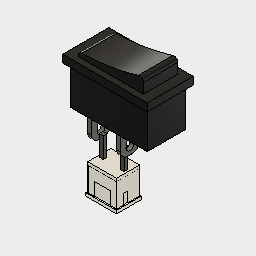
NewAssembly (Autodesk Fusion 360 archive; units mm, degrees)
design "Rocket Swith 15*10"
Autodesk Fusion 360 part; units mm, degrees
sketch "Sketch1" plane through (0, 0, 0) normal (0, 1, 0) x (1, 0, 0)
  line L0 (-10, 5) -> (10, 5)
  line L1 (10, 5) -> (10, -5)
  line L2 (10, -5) -> (-10, -5)
  line L3 (-10, -5) -> (-10, 5)
  dimension "d1" = 20
  dimension "d2" = 10
  dimension "d3" = 5
  dimension "d4" = 10
  measures "d1" distance of L0.start L0.end
  measures "d2" distance of L0.start L2.end
  measures "d3" distance of origin L0
  measures "d4" distance of origin L3
extrude "Extrude1" add sketch "Sketch1" along normal blind 10 makes body 1
sketch "Sketch2" plane through (0, 10, 0) normal (0, 1, 0) x (-1, 0, 0)
  line L0 (10, 5) -> (-10, 5)
  line L1 (-10, 5) -> (-10, -5)
  line L2 (-10, -5) -> (10, -5)
  line L3 (10, -5) -> (10, 5)
  line L4 (11, 6) -> (-11, 6)
  line L5 (-11, 6) -> (-11, -6)
  line L6 (-11, -6) -> (11, -6)
  line L7 (11, -6) -> (11, 6)
  dimension "d7" = 1
extrude "Extrude2" add sketch "Sketch2" along normal blind 2 contours L0 L1 L2 L3 | L4 L5 L6 L7 bodies 1
sketch "Sketch3" plane through (0, 12, 0) normal (0, 1, 0) x (-1, 0, 0)
  line L0 (11, -6) -> (11, 6)
  line L1 (11, 6) -> (-11, 6)
  line L2 (-11, 6) -> (-11, -6)
  line L3 (-11, -6) -> (11, -6)
  line L4 (-10, 5) -> (10, 5)
  line L5 (10, 5) -> (10, -5)
  line L6 (10, -5) -> (-10, -5)
  line L7 (-10, -5) -> (-10, 5)
  line L8 (-9.5, 4.5) -> (9.5, 4.5)
  line L9 (9.5, 4.5) -> (9.5, -4.5)
  line L10 (9.5, -4.5) -> (-9.5, -4.5)
  line L11 (-9.5, -4.5) -> (-9.5, 4.5)
  line L12 (9.5, -4.5) -> (8.5, -4.5)
  line L13 (8.5, -4.5) -> (8.5, 4.5)
  line L14 (8.5, 4.5) -> (9.5, 4.5)
  line L15 (9.5, 4.5) -> (9.5, -4.5)
  line L16 (-9.5, -4.5) -> (-8.5, -4.5)
  line L17 (-8.5, -4.5) -> (-8.5, 4.5)
  line L18 (-8.5, 4.5) -> (-9.5, 4.5)
  line L19 (-9.5, 4.5) -> (-9.5, -4.5)
  dimension "d14" = 0.5
  dimension "d15" = 1
  dimension "d16" = 1
  measures "d15" distance of L9.end L12.end
  measures "d16" distance of L10.end L16.end
extrude "Extrude3" add sketch "Sketch3" along normal blind 4 contours L8 L10 L13 L17 bodies 1
sketch "Sketch5" plane through (0, 0, 4.5) normal (0, 0, 1) x (1, 0, 0)
  line L0 (-8.5, 12) -> (8.5, 12)
  line L1 (8.5, 12) -> (8.5, 16)
  line L2 (8.5, 16) -> (-8.5, 16)
  line L3 (-8.5, 16) -> (-8.5, 12)
  spline S0 degree 5 poles (-8.5, 13.1583) (-8.1503, 13.1635) (-7.4519, 13.1784) (-6.4067, 13.2142) (-5.0183, 13.2895) (-3.2919, 13.4325) (-1.5755, 13.6289) (0.1301, 13.8829) (1.8245, 14.1971) (3.5081, 14.5689) (5.1818, 14.9942) (6.5133, 15.3737) (7.5081, 15.6789) (8.1697, 15.8915) (8.5, 16) knots 0 0 0 0 0 0 0.1 0.2 0.3 0.4 0.5 0.6 0.7 0.8 0.9 1 1 1 1 1 1
  line L4 (8.5, 12) -> (-8.5, 12)
  line L5 (-8.5, 12) -> (-8.5, 16)
  line L6 (-8.5, 16) -> (8.5, 16)
  line L7 (8.5, 16) -> (8.5, 12)
  point P0 (0.1376, 13.8996)
extrude "Extrude5" cut sketch "Sketch5" against normal blind 9 contours L2 L3 S0 L5 L6 bodies 1
fillet "Fillet1" radius 1 2 edges at (8.5, 16, 0) (-8.5, 13.1583, 0) on bodies 1
sketch "Sketch6" plane through (0, 0, 0) normal (0, -1, 0) x (1, 0, 0)
  line L0 (10, 5) -> (-10, 5)
  line L1 (-10, 5) -> (-10, -5)
  line L2 (-10, -5) -> (10, -5)
  line L3 (10, -5) -> (10, 5)
  line L4 (-8, 2.5) -> (-7, 2.5)
  line L5 (-7, 2.5) -> (-7, -2.5)
  line L6 (-7, -2.5) -> (-8, -2.5)
  line L7 (-8, -2.5) -> (-8, 2.5)
  line L8 (-0.5, 2.5) -> (0.5, 2.5)
  line L9 (0.5, 2.5) -> (0.5, -2.5)
  line L10 (0.5, -2.5) -> (-0.5, -2.5)
  line L11 (-0.5, -2.5) -> (-0.5, 2.5)
  dimension "d20" = 5
  dimension "d21" = 1
  dimension "d22" = 7
  dimension "d23" = 5
  dimension "d24" = 1
  dimension "d25" = 0.5
  dimension "d26" = 2.5
  measures "d20" distance of L4.start L6.end
  measures "d21" distance of L4.start L4.end
  measures "d22" distance of origin L5
  measures "d23" distance of L8.start L10.end
  measures "d24" distance of L8.start L8.end
  measures "d25" distance of origin L11
  measures "d26" distance of origin L8
extrude "Extrude6" add sketch "Sketch6" along normal blind 8 contours L4 L5 L6 L7 | L8 L9 L10 L11 bodies 1
sketch "Sketch7" plane through (0.5, 0, 0) normal (1, 0, 0) x (0, 0, -1)
  line L0 (2.5, 0) -> (-2.5, 0)
  line L1 (-2.5, 0) -> (-2.5, -8)
  line L2 (-2.5, -8) -> (2.5, -8)
  line L3 (2.5, -8) -> (2.5, 0)
  line L4 (1, -6) -> (1, -5)
  arc A0 (1, -5) -> (-1, -5) centre (0, -5) ccw
  line L5 (-1, -5) -> (-1, -6)
  arc A1 (-1, -6) -> (1, -6) centre (0, -6) ccw
  line L6 (0, -6) -> (0, -5) construction
  dimension "d29" = 1
  dimension "d30" = 1
  dimension "d31" = 5
  measures "d29" radius of A1
  measures "d30" distance of A1.centre A0.centre
  measures "d31" distance of origin A0.centre
extrude "Extrude7" cut sketch "Sketch7" against normal blind 8.5 contours L4 A0 L5 A1 bodies 1
fillet "Fillet2" radius 2 4 edges at (-7.5, -8, 2.5) (0, -8, 2.5) (0, -8, -2.5) (-7.5, -8, -2.5) on bodies 1
sketch "Sketch8" plane through (0, 0, -5) normal (0, 0, -1) x (-1, 0, 0)
  line L0 (-10, 0) -> (10, 0)
  line L1 (10, 0) -> (10, 10)
  line L2 (10, 10) -> (-10, 10)
  line L3 (-10, 10) -> (-10, 0)
  line L4 (7.5, -12) -> (0, -12)
  line L5 (0, -12) -> (0, -19)
  line L6 (0, -19) -> (7.5, -19)
  line L7 (7.5, -19) -> (7.5, -12)
  line L8 (6.5, -12) -> (7, -12)
  line L9 (7, -12) -> (7, -6)
  line L10 (7, -6) -> (6.5, -6)
  line L11 (6.5, -6) -> (6.5, -12)
  line L12 (0.5, -12) -> (1, -12)
  line L13 (1, -12) -> (1, -6)
  line L14 (1, -6) -> (0.5, -6)
  line L15 (0.5, -6) -> (0.5, -12)
  line L16 (0.5, 0) -> (0.5, -6)
  line L17 (7, 0) -> (7, -6)
  dimension "d35" = 7.5
  dimension "d36" = 7
  dimension "d37" = 12
  dimension "d38" = 0.5
  dimension "d39" = 0.5
  dimension "d40" = 6
  measures "d35" distance of L4.start L4.end
  measures "d36" distance of L4.start L6.end
  measures "d37" distance of origin L4
  measures "d38" distance of L13.end L14.end
  measures "d39" distance of L9.end L10.end
  measures "d40" distance of L8.end L9.end
extrude "Extrude8" add sketch "Sketch8" against normal blind 8 separate body contours L4 L5 L6 L7 L8 L12 makes body 2
extrude "Extrude9" cut 1 faces at (-2.8333, -16.6667, -5) along direction (0, 0, 1) blind 2 on bodies 2 bodies 2
sketch "Sketch9" plane through (0, -12, 0) normal (0, 1, 0) x (-1, 0, 0)
  line L0 (0, -3) -> (7.5, -3)
  line L1 (7.5, -3) -> (7.5, 3)
  line L2 (7.5, 3) -> (0, 3)
  line L3 (0, 3) -> (0, -3)
  line L4 (7, -0.5) -> (6, -0.5)
  line L5 (6, -0.5) -> (6, 0.5)
  line L6 (6, 0.5) -> (7, 0.5)
  line L7 (7, 0.5) -> (7, -0.5)
  line L8 (0.5, -0.5) -> (1.5, -0.5)
  line L9 (1.5, -0.5) -> (1.5, 0.5)
  line L10 (1.5, 0.5) -> (0.5, 0.5)
  line L11 (0.5, 0.5) -> (0.5, -0.5)
  line L12 (0.5, 1) -> (0.5, -1)
  line L13 (0.5, 1) -> (0.5, -1)
  line L14 (0.5, -0.5) -> (0.5, -2.5)
  line L15 (0.5, -0.5) -> (0.5, 0.5)
  line L16 (0.5, 2.5) -> (0.5, 0.5)
  line L17 (0.5, 2.5) -> (0.5, -2.5)
  line L18 (7, -2.5) -> (7, -0.5)
  line L19 (7, -2.5) -> (7, 2.5)
  line L20 (7, 0.5) -> (7, 2.5)
  line L21 (7, 0.5) -> (7, -0.5)
  line L22 (7, -1) -> (7, 1)
  line L23 (7, -1) -> (7, 1)
  point P0 (7, -2.5)
  dimension "d45" = 1
  dimension "d46" = 1
  dimension "d47" = 0.5
  dimension "d48" = 1
  measures "d45" distance of L8.start L8.end
  measures "d46" distance of L4.start L4.end
  measures "d47" distance of origin L8
  measures "d48" distance of L8.end L9.end
extrude "Extrude10" add sketch "Sketch9" along normal blind 5.326 contours L4 L5 L6 L7 L19 L21 L22 L23 | L8 L9 L10 L11 L12 L13 L15 L17 bodies 2
shell "Shell1" thickness 0.5 removed faces 1 at (-2.5, -19, -1) on bodies 2
sketch "Sketch10" plane through (0, 0, 0) normal (1, 0, 0) x (0, 0, -1)
  line L0 (3, -19) -> (3, -12)
  line L1 (3, -12) -> (-3, -12)
  line L2 (-3, -12) -> (-3, -19)
  line L3 (-3, -19) -> (3, -19)
  line L4 (-1.2673, -19) -> (0, -19)
  line L5 (0, -19) -> (0, -16.3604)
  line L6 (0, -16.3604) -> (-1.2673, -16.3604)
  line L7 (-1.2673, -16.3604) -> (-1.2673, -19)
extrude "Extrude11" cut sketch "Sketch10" against normal blind 7.5 contours L3 L4 L5 L6 L7 bodies 2
sketch "Sketch11" plane through (0, 0, 3) normal (0, 0, 1) x (1, 0, 0)
  line L0 (0, -19) -> (0, -12)
  line L1 (0, -12) -> (-7.5, -12)
  line L2 (-7.5, -12) -> (-7.5, -19)
  line L3 (-7.5, -19) -> (0, -19)
  line L4 (-5.8268, -19) -> (-1.5543, -19)
  line L5 (-1.5543, -19) -> (-1.5543, -15.6198)
  line L6 (-1.5543, -15.6198) -> (-5.8268, -15.6198)
  line L7 (-5.8268, -15.6198) -> (-5.8268, -19)
extrude "Extrude12" cut sketch "Sketch11" against normal blind 5.5 contours L3 L4 L5 L6 L7 bodies 2
sketch "Sketch12" plane through (0, -19, 0) normal (0, -1, 0) x (1, 0, 0)
  line L0 (0, 0) -> (-0.5, 0)
  line L1 (-0.5, 0) -> (-0.5, -2.5)
  line L2 (-0.5, -2.5) -> (-7, -2.5)
  line L3 (-7, -2.5) -> (-7, 0)
  line L4 (-7, 0) -> (-7.5, 0)
  line L5 (-7.5, 0) -> (-7.5, -3)
  line L6 (-7.5, -3) -> (0, -3)
  line L7 (0, -3) -> (0, 0)
  line L8 (-7.75, 3.25) -> (0.25, 3.25)
  line L9 (0.25, 3.25) -> (0.25, -3.25)
  line L10 (0.25, -3.25) -> (-7.75, -3.25)
  line L11 (-7.75, -3.25) -> (-7.75, 3.25)
  line L12 (0, 1.2673) -> (0, 3)
  line L13 (-7.5, 3) -> (-5.8268, 3)
  dimension "d56" = 8
  dimension "d57" = 6.5
  dimension "d58" = 0.25
  dimension "d59" = 0.25
  measures "d56" distance of L8.start L8.end
  measures "d57" distance of L8.start L10.end
  measures "d58" distance of L9 L12
  measures "d59" distance of L8 L13
extrude "Extrude13" add sketch "Sketch12" along normal blind 0.8 separate body contours L0 L1 L2 L3 L4 L5 L6 L7 | L8 L9 L10 L11 makes body 3
sketch "Sketch13" plane through (0, -19, 0) normal (0, 1, 0) x (-1, 0, 0)
  line L0 (-0.25, -3.25) -> (7.75, -3.25)
  line L1 (7.75, -3.25) -> (7.75, 3.25)
  line L2 (7.75, 3.25) -> (-0.25, 3.25)
  line L3 (-0.25, 3.25) -> (-0.25, -3.25)
  line L4 (7.35, -2.9) -> (0.15, -2.9)
  line L5 (0.15, -2.9) -> (0.15, 2.9)
  line L6 (0.15, 2.9) -> (7.35, 2.9)
  line L7 (7.35, 2.9) -> (7.35, -2.9)
  dimension "d62" = 7.2
  dimension "d63" = 5.8
  dimension "d64" = 0.4
  dimension "d65" = 0.35
  measures "d62" distance of L4.start L4.end
  measures "d63" distance of L4.start L6.end
  measures "d64" distance of L3 L5
  measures "d65" distance of L0 L4
extrude "Extrude14" add sketch "Sketch13" along normal blind 6.142 contours L4 L5 L6 L7 bodies 3
sketch "Sketch14" plane through (0, -19.8, 0) normal (0, -1, 0) x (1, 0, 0)
  line L0 (-7.75, -3.25) -> (0.25, -3.25)
  line L1 (0.25, -3.25) -> (0.25, 3.25)
  line L2 (0.25, 3.25) -> (-7.75, 3.25)
  line L3 (-7.75, 3.25) -> (-7.75, -3.25)
  circle A0 centre (-5.25, 0) radius 0.75
  circle A1 centre (-2.25, 0) radius 0.75
  dimension "d68" = 1.5
  dimension "d69" = 1.5
  dimension "d70" = 3
  dimension "d71" = 2.5
  measures "d68" diameter of A0
  measures "d69" diameter of A1
  measures "d70" distance of A0.centre A1.centre
  measures "d71" distance of L1 A1.centre
extrude "Extrude15" add sketch "Sketch14" along normal blind 0.5 contours A0 | A1 bodies 3

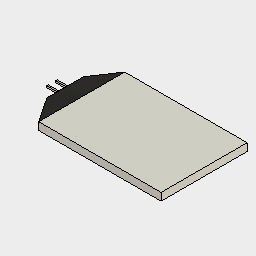
design "Stage Holder"
Autodesk Fusion 360 part; units mm, degrees
sketch "Sketch1" plane through (0, 0, 0) normal (0, 0, 1) x (1, 0, 0)
  line L0 (-21, 13) -> (21, 13)
  line L1 (21, 13) -> (21, -13)
  line L2 (21, -13) -> (-21, -13)
  line L3 (-21, -13) -> (-21, 13)
  line L4 (-16, 13) -> (-16, -13)
  line L5 (-16, 13) -> (-21, 5.5)
  line L6 (-16, -13) -> (-21, -5.5)
  line L7 (-21, 0) -> (-18.5, 0)
  dimension "d1" = 42
  dimension "d2" = 26
  dimension "d3" = 13
  dimension "d4" = 21
  dimension "d5" = 37
  dimension "d6" = 11
  dimension "d7" = 5.5
  measures "d1" distance of L0.start L0.end
  measures "d2" distance of L0.start L2.end
  measures "d3" distance of origin L0
  measures "d4" distance of origin L3
  measures "d5" distance of L1 L4
  measures "d6" distance of L5.end L6.end
  measures "d7" distance of L5.end L7.end
extrude "Extrude1" add sketch "Sketch1" along normal blind 2.3 contours L0 L1 L2 L4 | L3 L4 L5 L6 makes body 1
sketch "Sketch2" plane through (-21, 0, 0) normal (-1, 0, 0) x (0, -1, 0)
  line L0 (-5.5, 0) -> (5.5, 0)
  line L1 (5.5, 0) -> (5.5, 2.3)
  line L2 (5.5, 2.3) -> (-5.5, 2.3)
  line L3 (-5.5, 2.3) -> (-5.5, 0)
  line L4 (-1.575, 1.5) -> (-1.075, 1.5)
  line L5 (-1.075, 1.5) -> (-1.075, 1)
  line L6 (-1.075, 1) -> (-1.575, 1)
  line L7 (-1.575, 1) -> (-1.575, 1.5)
  line L8 (1.075, 1.5) -> (1.575, 1.5)
  line L9 (1.575, 1.5) -> (1.575, 1)
  line L10 (1.575, 1) -> (1.075, 1)
  line L11 (1.075, 1) -> (1.075, 1.5)
  dimension "d11" = 3.15
  dimension "d12" = 0.5
  dimension "d13" = 0.5
  dimension "d14" = 1.575
  dimension "d15" = 1
  dimension "d16" = 0.5
  measures "d11" distance of L7 L9
  measures "d12" distance of L4.start L4.end
  measures "d13" distance of L8.start L8.end
  measures "d14" distance of origin L9
  measures "d15" distance of L0 L10
  measures "d16" distance of L8.end L9.end
extrude "Extrude2" add sketch "Sketch2" along normal blind 4 contours L4 L5 L6 L7 | L8 L9 L10 L11 bodies 1
ref_plane "WorkPlane1" through (-16, 0, 1.15) normal (-1, 0, 0) x (0, -1, 0)
split "Split1" by plane through (-16, 0, 1.15) normal (-1, 0, 0) bodies 1 makes body 2 at (-17.6667, -1.8333, 0)
equation "d3 = d2 / 2"
equation "d4 = d1 / 2"
equation "d7 = d6 / 2"
equation "d14 = d11 / 2"

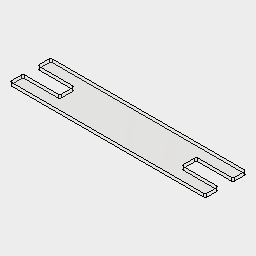
design "Light Holder 2mm"
Autodesk Fusion 360 part; units mm, degrees
sketch "Sketch1" plane through (0, 0, 0) normal (0, 0, 1) x (1, 0, 0)
  line L0 (-60, 12.5) -> (60, 12.5)
  line L1 (60, 12.5) -> (60, 4.5)
  line L2 (60, 4.5) -> (-60, 4.5)
  line L3 (-60, 4.5) -> (-60, 12.5)
  line L4 (-60, -4.5) -> (60, -4.5)
  line L5 (60, -4.5) -> (60, -12.5)
  line L6 (60, -12.5) -> (-60, -12.5)
  line L7 (-60, -12.5) -> (-60, -4.5)
  line L8 (-37.5, 4.5) -> (37.5, 4.5)
  line L9 (37.5, 4.5) -> (37.5, -4.5)
  line L10 (37.5, -4.5) -> (-37.5, -4.5)
  line L11 (-37.5, -4.5) -> (-37.5, 4.5)
  dimension "d24" = 120
  dimension "d25" = 8
  dimension "d26" = 8
  dimension "d27" = 25
  dimension "d28" = 75
  dimension "d34" = 60
  dimension "d35" = 12.5
  dimension "d38" = 37.5
  measures "d24" distance of L0.start L0.end
  measures "d25" distance of L0.start L2.end
  measures "d26" distance of L4.start L6.end
  measures "d27" distance of L0 L6
  measures "d28" distance of L8.start L8.end
  measures "d34" distance of origin L3
  measures "d35" distance of origin L0
  measures "d38" distance of origin L9
extrude "Extrude1" add sketch "Sketch1" along normal blind 2
fillet "Fillet1" radius 1 12 edges at (-60, 12.5, 1) (-60, 4.5, 1) (-60, -4.5, 1) (-60, -12.5, 1) (-37.5, 4.5, 1) (-37.5, -4.5, 1) (60, -12.5, 1) (60, -4.5, 1) (37.5, 4.5, 1) (37.5, -4.5, 1) (60, 4.5, 1) (60, 12.5, 1)
equation "d26 = d25"
equation "d34 = d24 / 2"
equation "d35 = d27 / 2"
equation "d38 = d28 / 2"

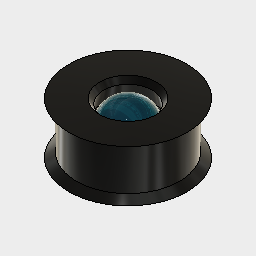
design "Lens Clip"
Autodesk Fusion 360 part; units mm, degrees
sketch "Sketch2" plane through (0, 0, 0) normal (0, 0, 1) x (1, 0, 0)
sphere "SpherePrimitive2" add diameter 2 placed x (1, 0, 0) y (0, 1, 0) z (0, 0, 1) at (0, 0, 0) makes body 1
sketch "Sketch3" plane through (0, 0, 0) normal (0, 1, 0) x (1, 0, 0)
  circle A0 centre (0, 0) radius 1.1
  line L0 (-2.3, -1) -> (2.3, -1)
  line L1 (2.3, -1) -> (2.3, 1)
  line L2 (2.3, 1) -> (-2.3, 1)
  line L3 (-2.3, 1) -> (-2.3, -1)
  line L4 (-0.9, -1) -> (-1.0724, -0.2448)
  line L5 (0.9, -1) -> (1.0724, -0.2448)
  line L6 (0, -1) -> (0, 1)
  line L7 (-2, -0.8) -> (2, -0.8)
  line L8 (2, -0.8) -> (2, 0.8)
  line L9 (2, 0.8) -> (-2, 0.8)
  line L10 (-2, 0.8) -> (-2, -0.8)
  line L11 (2, -0.8) -> (2.3, -1)
  line L12 (2, 0.8) -> (2.3, 1)
  dimension "d3" = 2.2
  dimension "d4" = 4.6
  dimension "d5" = 2.3
  dimension "d6" = 2
  dimension "d7" = 1
  dimension "d8" = 1.4
  dimension "d9" = 1.4
  dimension "d11" = 4
  dimension "d12" = 1.6
  dimension "d13" = 0.8
  dimension "d14" = 2
  measures "d3" diameter of A0
  measures "d4" distance of L0.start L0.end
  measures "d5" distance of A0.centre L3
  measures "d6" distance of L0.start L2.end
  measures "d7" distance of A0.centre L0
  measures "d8" distance of L1 L5.start
  measures "d9" distance of L3 L4.start
  measures "d11" distance of L7.start L7.end
  measures "d12" distance of L7.start L9.end
  measures "d13" distance of A0.centre L7
  measures "d14" distance of A0.centre L8
revolve "Revolve1" add sketch "Sketch3" angle 360 about axis through (0, 0, 1) along (0, 0, -1) separate body contours A0 L5 L7 L8 L9 | L0 L5 L7 L11 | A0 L2 L9 L12 makes body 2
chamfer "Chamfer1" distance 0.2 angle 45 1 edges at (-0.8391, -0.3255, 1) on bodies 2
equation "d5 = d4 / 2"
equation "d7 = d6 / 2"
equation "d9 = d8"
